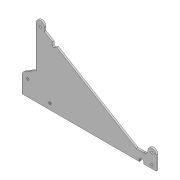
# Autodesk Inventor part: 5linerail
Saved by Autodesk Inventor 2020 (Build 240168000, 168)
## iProperties
Created: 2021-06-11
Part Number: 5linerail
Material: Generic
Document SubType Name: Modeling
Designer: Aidan Lee
Density: 1 g/cm^3
Appearance: Default
Author: Aidan Lee
Autodesk Inventor part; units mm, degrees
ref_plane "YZ Plane" through (0, 0, 0) normal (1, 0, 0) x (0, 1, 0)
ref_plane "XZ Plane" through (0, 0, 0) normal (0, 1, 0) x (-1, 0, 0)
ref_plane "XY Plane" through (0, 0, 0) normal (0, 0, 1) x (1, 0, 0)
sketch "Sketch3" plane through (0, 0, 0) normal (0, 0, 1) x (1, 0, 0)
  circle A0 centre (367.816, 50) radius 50 construction
  line L0 (367.816, 0) -> (512.7041, 0) construction
  line L1 (367.816, 50) -> (512.7041, 50) construction
  line L2 (367.816, 100) -> (512.7041, 100) construction
  line L3 (367.816, 50) -> (342.816, 6.6987) construction
  line L4 (367.816, 50) -> (324.5147, 25) construction
  line L5 (367.816, 50) -> (324.5147, 75) construction
  line L6 (342.816, 93.3013) -> (367.816, 50) construction
  line L7 (392.816, 93.3013) -> (367.816, 50) construction
  line L8 (411.1173, 75) -> (367.816, 50) construction
  line L9 (411.1173, 25) -> (367.816, 50) construction
  line L10 (392.816, 6.6987) -> (367.816, 50) construction
  line L11 (367.816, 0) -> (367.816, 100) construction
  line L12 (417.816, 50) -> (367.816, 50) construction
  line L13 (341.6361, 0) -> (341.6361, 100) construction
  line L14 (315.4561, 0) -> (315.4561, 100) construction
  line L15 (289.2762, 0) -> (289.2762, 100) construction
  line L16 (263.0963, 0) -> (263.0963, 100) construction
  line L17 (236.9163, 0) -> (236.9163, 100) construction
  line L18 (210.7364, 0) -> (210.7364, 100) construction
  line L19 (184.5564, 0) -> (184.5564, 100) construction
  line L20 (158.3765, 0) -> (158.3765, 100) construction
  circle A1 centre (315.4561, 50) radius 50 construction
  circle A2 centre (341.6361, 50) radius 50 construction
  circle A3 centre (289.2762, 50) radius 50 construction
  circle A4 centre (263.0963, 50) radius 50 construction
  circle A5 centre (236.9163, 50) radius 50 construction
  circle A6 centre (210.7364, 50) radius 50 construction
  line L21 (392.816, 6.6987) -> (512.7041, 6.6987) construction
  line L22 (411.1173, 25) -> (512.7041, 25) construction
  line L23 (411.1173, 75) -> (512.7041, 75) construction
  line L24 (411.1173, 75) -> (512.7041, 75) construction
  line L25 (392.816, 93.3013) -> (512.7041, 93.3013) construction
  line L26 (358.7574, 75) -> (339.2762, 50) construction
  line L27 (339.2762, 50) -> (306.3975, 25) construction
  line L28 (306.3975, 25) -> (261.9163, 6.6987) construction
  line L29 (261.9163, 6.6987) -> (210.7364, 0) construction
  line L30 (105.3682, -12.9392) -> (105.3682, 124.4333) construction
  line L31 (21.25, 0) -> (21.25, 12)
  line L32 (35.45, 12) -> (35.45, -11.8433)
  arc A7 (0, 0) -> (6.625, -9.8433) centre (10.625, 0) ccw
  arc A8 (14.625, -9.8433) -> (21.25, 0) centre (10.625, 0) ccw
  line L33 (35.45, -11.8433) -> (14.625, -11.8433)
  line L34 (6.625, -11.8433) -> (-195.0796, -11.8433)
  circle A9 centre (-144.26, 100.8473) radius 12.875 construction
  line L35 (6.625, -11.8433) -> (6.625, -9.8433)
  line L36 (14.625, -11.8433) -> (14.625, -9.8433)
  line L37 (411.1173, 75) -> (158.3765, 75) construction
  line L38 (367.816, 100) -> (158.3765, 100) construction
  line L39 (417.816, 50) -> (158.3765, 50) construction
  line L40 (411.1173, 25) -> (158.3765, 25) construction
  line L41 (392.816, 6.6987) -> (158.3765, 6.6987) construction
  line L42 (392.816, 93.3013) -> (158.3765, 93.3013) construction
  line L43 (358.7574, 75) -> (366.6361, 93.3013) construction
  line L44 (366.6361, 93.3013) -> (367.816, 100) construction
  spline S0 degree 4 poles (-157.0796, 100) (-157.0796, 88.9946) (-147.011, 72.6811) (-131.8577, 48.7932) (-88.4777, 17.6268) (-50.0176, 3.937) (-18.8717, 0) (0, 0) knots 0 0 0 0 0 0.264547 0.457223 0.66608 1 1 1 1 1
  line L45 (-157.0796, 100) -> (-157.0796, 38) construction
  line L46 (0, 0) -> (-157.0796, 0) construction
  line L47 (-144.26, 100.8473) -> (-157.135, 100.8473) construction
  circle A10 centre (-146.4546, 100) radius 10.625 construction
  line L48 (-146.4546, 100) -> (-157.0796, 100) construction
  line L49 (-141.0754, 84.4005) -> (-135.6205, 93.5183) construction
  line L50 (-141.0796, 132.0528) -> (-171.0796, 149.3733) construction
  line L51 (-171.0796, 149.3733) -> (-201.0796, 132.0528) construction
  line L52 (-141.0754, 84.4005) -> (-99.2801, 84.4005) construction
  line L53 (-201.0796, 132.0528) -> (-201.0796, 97.4118) construction
  line L54 (-201.0796, 97.4118) -> (-171.0796, 80.0913) construction
  line L55 (0, 0) -> (-157.0796, 93.9753) construction
  line L56 (-135.6205, 93.5183) -> (-137.3368, 94.5451) construction
  line L57 (-137.3368, 94.5451) -> (-143.2815, 84.6085) construction
  line L58 (-137.3368, 94.5451) -> (-171.0796, 114.7323) construction
  line L59 (-201.0796, 132.0528) -> (-171.0796, 114.7323) construction
  arc A11 (-137.3368, 94.5451) -> (-144.7045, 143.8948) centre (-171.0796, 114.7323) ccw construction
  arc A12 (-142.7917, 85.4273) -> (-147.1443, 147.6882) centre (-171.0796, 114.7323) ccw construction
  line L60 (-171.0796, 80.0913) -> (-171.0796, 35)
  circle A13 centre (-171.0796, 114.7323) radius 2.5 construction
  arc A14 (-167.4345, 120.8251) -> (-174.7248, 108.6394) centre (-171.0796, 114.7323) ccw construction
  line L61 (-167.4345, 120.8251) -> (-157.0796, 114.6302) construction
  line L62 (-171.0796, 80.0913) -> (-171.0796, 106.4587)
  line L63 (-171.0796, 106.4587) -> (-174.7248, 108.6394) construction
  line L64 (-171.0796, 35) -> (-191.5296, 23.1932)
  arc A15 (-191.5296, 23.1932) -> (-195.0796, 17.0444) centre (-187.9796, 17.0444) ccw
  line L65 (-195.0796, 17.0444) -> (-195.0796, -11.8433)
  arc A16 (35.45, 12) -> (21.25, 12) centre (28.35, 12) ccw
  line L66 (-157.0796, 114.6302) -> (-157.0796, 99.9865) construction
  circle A17 centre (-164.0796, 103.4587) radius 2
  line L67 (-171.0796, 103.4587) -> (-157.0796, 103.4587) construction
  circle A18 centre (-185.1284, 15.3983) radius 2
  line L68 (-185.1284, 15.3983) -> (-194.1284, 20.5944) construction
  circle A19 centre (-6, -5.9217) radius 2
  line L69 (-6, -11.8433) -> (-6, 0) construction
  circle A20 centre (28.35, 12) radius 2
  circle A21 centre (28.35, -5.9217) radius 2
  line L70 (-167.4345, 320.8251) -> (-157.0796, 314.6302) construction
  arc A22 (-167.4345, 320.8251) -> (-174.7248, 308.6394) centre (-171.0796, 314.7323) ccw construction
  circle A23 centre (-171.0796, 314.7323) radius 2.5 construction
  line L71 (-171.0796, 280.0913) -> (-171.0796, 306.4587)
  line L72 (-171.0796, 306.4587) -> (-174.7248, 308.6394) construction
  line L73 (-157.0796, 314.6302) -> (-157.0796, 299.9865) construction
  circle A24 centre (-164.0796, 303.4587) radius 2
  spline S1 degree 4 poles (-157.0796, 300) (-157.0796, 288.9946) (-147.0234, 272.6841) (-124.1789, 236.7977) (-70.8039, 208.0704) (-31.8865, 200.2943) (0, 200) knots 0 0 0 0 0 0.264547 0.457223 1 1 1 1 1 construction
  line L74 (-157.0796, 300) -> (-157.0796, 238) construction
  arc A25 (0, 200) -> (6.625, 190.1567) centre (10.625, 200) ccw
  line L75 (35.45, 212) -> (35.45, 188.1567)
  circle A26 centre (28.35, 212) radius 2
  circle A27 centre (28.35, 194.0783) radius 2
  arc A28 (35.45, 212) -> (21.25, 212) centre (28.35, 212) ccw
  line L76 (21.25, 200) -> (21.25, 212)
  line L77 (35.45, 188.1567) -> (14.625, 188.1567)
  arc A29 (14.625, 190.1567) -> (21.25, 200) centre (10.625, 200) ccw
  line L78 (14.625, 188.1567) -> (14.625, 190.1567)
  line L79 (-185.1284, 215.3983) -> (-194.1284, 220.5944) construction
  arc A30 (-191.5296, 223.1932) -> (-195.0796, 217.0444) centre (-187.9796, 217.0444) ccw
  line L80 (-195.0796, 217.0444) -> (-195.0796, 188.1567)
  line L81 (-171.0796, 235) -> (-191.5296, 223.1932)
  circle A31 centre (-185.1284, 215.3983) radius 2
  line L82 (-171.0796, 280.0913) -> (-171.0796, 235)
  line L83 (6.625, 188.1567) -> (-195.0796, 188.1567)
  line L84 (6.625, 188.1567) -> (6.625, 190.1567)
  line L85 (-137.3368, 294.5451) -> (-143.2815, 284.6085) construction
  line L86 (-141.0754, 284.4005) -> (-135.6205, 293.5183) construction
  line L87 (0, 200) -> (-157.0796, 293.9753)
  line L88 (-167.4345, 520.8251) -> (-157.0796, 514.6302) construction
  arc A32 (-167.4345, 520.8251) -> (-174.7248, 508.6394) centre (-171.0796, 514.7323) ccw construction
  circle A33 centre (-171.0796, 514.7323) radius 2.5 construction
  line L89 (-171.0796, 480.0913) -> (-171.0796, 506.4587)
  line L90 (-171.0796, 506.4587) -> (-174.7248, 508.6394) construction
  line L91 (-157.0796, 514.6302) -> (-157.0796, 499.9865) construction
  circle A34 centre (-164.0796, 503.4587) radius 2
  spline S2 degree 4 poles (-157.0796, 500) (-157.0796, 488.9946) (-147.0234, 472.6841) (-124.1789, 436.7977) (-70.8039, 408.0704) (-31.8865, 400.2943) (0, 400) knots 0 0 0 0 0 0.264547 0.457223 1 1 1 1 1 construction
  line L92 (-157.0796, 500) -> (-157.0796, 438)
  arc A35 (0, 400) -> (6.625, 390.1567) centre (10.625, 400) ccw
  line L93 (35.45, 412) -> (35.45, 388.1567)
  circle A36 centre (28.35, 412) radius 2
  circle A37 centre (28.35, 394.0783) radius 2
  arc A38 (35.45, 412) -> (21.25, 412) centre (28.35, 412) ccw
  line L94 (21.25, 400) -> (21.25, 412)
  line L95 (35.45, 388.1567) -> (14.625, 388.1567)
  arc A39 (14.625, 390.1567) -> (21.25, 400) centre (10.625, 400) ccw
  line L96 (14.625, 388.1567) -> (14.625, 390.1567)
  line L97 (-185.1284, 415.3983) -> (-194.1284, 420.5944) construction
  arc A40 (-191.5296, 423.1932) -> (-195.0796, 417.0444) centre (-187.9796, 417.0444) ccw
  line L98 (-195.0796, 417.0444) -> (-195.0796, 388.1567)
  line L99 (-171.0796, 435) -> (-191.5296, 423.1932)
  circle A41 centre (-185.1284, 415.3983) radius 2
  line L100 (-171.0796, 480.0913) -> (-171.0796, 435)
  line L101 (6.625, 388.1567) -> (-195.0796, 388.1567)
  line L102 (6.625, 388.1567) -> (6.625, 390.1567)
  line L103 (-137.3368, 494.5451) -> (-143.2815, 484.6085) construction
  line L104 (-141.0754, 484.4005) -> (-135.6205, 493.5183) construction
  line L105 (0, 400) -> (-157.0796, 493.9753) construction
  line L106 (-467.4345, 120.8251) -> (-457.0796, 114.6302) construction
  arc A42 (-467.4345, 120.8251) -> (-474.7248, 108.6394) centre (-471.0796, 114.7323) ccw construction
  circle A43 centre (-471.0796, 114.7323) radius 2.5 construction
  line L107 (-471.0796, 80.0913) -> (-471.0796, 106.4587)
  line L108 (-471.0796, 106.4587) -> (-474.7248, 108.6394) construction
  line L109 (-457.0796, 114.6302) -> (-457.0796, 99.9865) construction
  circle A44 centre (-464.0796, 103.4587) radius 2
  spline S3 degree 4 poles (-457.0796, 100) (-457.0796, 88.9946) (-447.0234, 72.6841) (-424.1789, 36.7977) (-370.8039, 8.0704) (-331.8865, 0.2943) (-300, 0) knots 0 0 0 0 0 0.264547 0.457223 1 1 1 1 1 construction
  line L110 (-457.0796, 100) -> (-457.0796, 38) construction
  arc A45 (-300, 0) -> (-293.375, -9.8433) centre (-289.375, 0) ccw construction
  line L111 (-264.55, 12) -> (-264.55, -11.8433)
  circle A46 centre (-271.65, 12) radius 2
  circle A47 centre (-271.65, -5.9217) radius 2
  arc A48 (-264.55, 12) -> (-278.75, 12) centre (-271.65, 12) ccw
  line L112 (-278.75, 0) -> (-278.75, 12) construction
  line L113 (-264.55, -11.8433) -> (-285.375, -11.8433)
  arc A49 (-285.375, -9.8433) -> (-278.75, 0) centre (-289.375, 0) ccw construction
  line L114 (-285.375, -11.8433) -> (-285.375, -9.8433) construction
  line L115 (-485.1284, 15.3983) -> (-494.1284, 20.5944) construction
  arc A50 (-491.5296, 23.1932) -> (-495.0796, 17.0444) centre (-487.9796, 17.0444) ccw
  line L116 (-495.0796, 17.0444) -> (-495.0796, -11.8433)
  line L117 (-471.0796, 35) -> (-491.5296, 23.1932)
  circle A51 centre (-485.1284, 15.3983) radius 2
  line L118 (-471.0796, 80.0913) -> (-471.0796, 35)
  line L119 (-293.375, -11.8433) -> (-495.0796, -11.8433)
  line L120 (-293.375, -11.8433) -> (-293.375, -9.8433) construction
  line L121 (-437.3368, 94.5451) -> (-443.2815, 84.6085) construction
  line L122 (-441.0754, 84.4005) -> (-435.6205, 93.5183) construction
  line L123 (-300, 0) -> (-457.0796, 93.9753) construction
  line L124 (-467.4345, 320.8251) -> (-457.0796, 314.6302) construction
  arc A52 (-467.4345, 320.8251) -> (-474.7248, 308.6394) centre (-471.0796, 314.7323) ccw construction
  circle A53 centre (-471.0796, 314.7323) radius 2.5 construction
  line L125 (-471.0796, 280.0913) -> (-471.0796, 306.4587)
  line L126 (-471.0796, 306.4587) -> (-474.7248, 308.6394) construction
  line L127 (-457.0796, 314.6302) -> (-457.0796, 299.9865) construction
  circle A54 centre (-464.0796, 303.4587) radius 2
  spline S4 degree 4 poles (-457.0796, 300) (-457.0796, 288.9946) (-447.0234, 272.6841) (-424.1789, 236.7977) (-370.8039, 208.0704) (-331.8865, 200.2943) (-300, 200) knots 0 0 0 0 0 0.264547 0.457223 1 1 1 1 1 construction
  line L128 (-457.0796, 300) -> (-457.0796, 238) construction
  arc A55 (-300, 200) -> (-293.375, 190.1567) centre (-289.375, 200) ccw construction
  line L129 (-264.55, 212) -> (-264.55, 188.1567)
  circle A56 centre (-271.65, 212) radius 2
  circle A57 centre (-271.65, 194.0783) radius 2
  arc A58 (-264.55, 212) -> (-278.75, 212) centre (-271.65, 212) ccw
  line L130 (-278.75, 200) -> (-278.75, 212) construction
  line L131 (-264.55, 188.1567) -> (-285.375, 188.1567)
  arc A59 (-285.375, 190.1567) -> (-278.75, 200) centre (-289.375, 200) ccw construction
  line L132 (-285.375, 188.1567) -> (-285.375, 190.1567) construction
  line L133 (-485.1284, 215.3983) -> (-494.1284, 220.5944) construction
  arc A60 (-491.5296, 223.1932) -> (-495.0796, 217.0444) centre (-487.9796, 217.0444) ccw
  line L134 (-495.0796, 217.0444) -> (-495.0796, 188.1567)
  line L135 (-471.0796, 235) -> (-491.5296, 223.1932)
  circle A61 centre (-485.1284, 215.3983) radius 2
  line L136 (-471.0796, 280.0913) -> (-471.0796, 235)
  line L137 (-293.375, 188.1567) -> (-495.0796, 188.1567)
  line L138 (-293.375, 188.1567) -> (-293.375, 190.1567) construction
  line L139 (-437.3368, 294.5451) -> (-443.2815, 284.6085) construction
  line L140 (-441.0754, 284.4005) -> (-435.6205, 293.5183) construction
  line L141 (-300, 200) -> (-457.0796, 293.9753) construction
  line L142 (-467.4345, 520.8251) -> (-457.0796, 514.6302)
  arc A62 (-467.4345, 520.8251) -> (-474.7248, 508.6394) centre (-471.0796, 514.7323) ccw
  circle A63 centre (-471.0796, 514.7323) radius 2.5
  line L143 (-471.0796, 480.0913) -> (-471.0796, 506.4587)
  line L144 (-471.0796, 506.4587) -> (-474.7248, 508.6394)
  line L145 (-457.0796, 514.6302) -> (-457.0796, 499.9865)
  circle A64 centre (-464.0796, 503.4587) radius 2
  spline S5 degree 4 poles (-457.0796, 500) (-457.0796, 488.9946) (-447.0234, 472.6841) (-424.1789, 436.7977) (-370.8039, 408.0704) (-331.8865, 400.2943) (-300, 400) knots 0 0 0 0 0 0.264547 0.457223 1 1 1 1 1 construction
  line L146 (-457.0796, 500) -> (-457.0796, 438) construction
  arc A65 (-300, 400) -> (-293.375, 390.1567) centre (-289.375, 400) ccw construction
  line L147 (-264.55, 412) -> (-264.55, 388.1567) construction
  circle A66 centre (-271.65, 412) radius 2
  circle A67 centre (-271.65, 394.0783) radius 2
  arc A68 (-264.55, 412) -> (-278.75, 412) centre (-271.65, 412) ccw
  line L148 (-278.75, 400) -> (-278.75, 412) construction
  line L149 (-264.55, 388.1567) -> (-285.375, 388.1567)
  arc A69 (-285.375, 390.1567) -> (-278.75, 400) centre (-289.375, 400) ccw construction
  line L150 (-285.375, 388.1567) -> (-285.375, 390.1567) construction
  line L151 (-485.1284, 415.3983) -> (-494.1284, 420.5944) construction
  arc A70 (-491.5296, 423.1932) -> (-495.0796, 417.0444) centre (-487.9796, 417.0444) ccw
  line L152 (-495.0796, 417.0444) -> (-495.0796, 388.1567) construction
  line L153 (-471.0796, 435) -> (-491.5296, 423.1932)
  circle A71 centre (-485.1284, 415.3983) radius 2
  line L154 (-471.0796, 480.0913) -> (-471.0796, 435)
  line L155 (-293.375, 388.1567) -> (-495.0796, 388.1567)
  line L156 (-293.375, 388.1567) -> (-293.375, 390.1567) construction
  line L157 (-437.3368, 494.5451) -> (-443.2815, 484.6085) construction
  line L158 (-441.0754, 484.4005) -> (-435.6205, 493.5183) construction
  line L159 (-300, 400) -> (-457.0796, 493.9753) construction
  line L160 (-435.4304, 87.048) -> (-430.3073, 83.9831)
  line L161 (-430.3073, 83.9831) -> (-430.3073, 78.0131)
  line L162 (-457.0796, 100) -> (-443.128, 91.6532)
  line L163 (-443.2208, 85.684) -> (-443.128, 91.6532)
  line L164 (-440.6463, 84.1438) -> (-435.4304, 87.048)
  line L165 (-440.6463, 84.1438) -> (-443.2208, 85.684)
  line L166 (-430.3073, 78.0131) -> (-436.0283, 74.7101)
  line L167 (-436.0283, 74.7101) -> (-436.0283, 68.1041)
  spline S6 degree 4 poles (-439.3753, 72.7777) (-420.1522, 45.3403) (-398.6357, 22.4496) (-337.1208, 4.2654) (-300, 5.1701) knots 0 0 0 0 0 1 1 1 1 1
  line L168 (-293.375, -11.8433) -> (-285.375, -11.8433)
  line L169 (-157.0796, 293.9753) -> (-157.0796, 300)
  line L170 (-293.375, 188.1567) -> (-285.375, 188.1567)
  arc A72 (-157.0796, 438) -> (-119.0796, 400) centre (-119.0796, 438) ccw
  line L171 (-119.0796, 400) -> (0, 400)
  line L172 (-457.0796, 500) -> (-457.0796, 438) construction
  line L173 (-419.0796, 400) -> (-300, 400) construction
  arc A73 (-457.0796, 438) -> (-419.0796, 400) centre (-419.0796, 438) ccw construction
  line L174 (-457.0796, 300) -> (-443.128, 291.6532)
  line L175 (-443.2208, 285.684) -> (-443.128, 291.6532)
  line L176 (-440.6463, 284.1438) -> (-443.2208, 285.684)
  line L177 (-440.6463, 284.1438) -> (-435.4304, 287.048)
  line L178 (-435.4304, 287.048) -> (-430.3073, 283.9831)
  line L179 (-430.3073, 283.9831) -> (-430.3073, 278.0131) construction
  line L180 (-430.3073, 278.0131) -> (-436.0283, 274.7101) construction
  line L181 (-457.0796, 500) -> (-443.128, 491.6532)
  line L182 (-443.2208, 485.684) -> (-443.128, 491.6532)
  line L183 (-440.6463, 484.1438) -> (-443.2208, 485.684)
  line L184 (-440.6463, 484.1438) -> (-435.4304, 487.048)
  line L185 (-435.4304, 487.048) -> (-430.3073, 483.9831)
  line L186 (-430.3073, 483.9831) -> (-430.3073, 478.0131)
  line L187 (-430.3073, 478.0131) -> (-436.0283, 474.7101)
  line L188 (-430.3073, 283.9831) -> (-298.5715, 205.1701)
  line L189 (-293.375, 388.1567) -> (-285.375, 388.1567)
  line L190 (-300, 5.1701) -> (-285.5799, 5.1701)
  arc A74 (-285.5799, 5.1701) -> (-278.75, 12) centre (-285.5799, 12) ccw
  line L191 (-298.5715, 205.1701) -> (-285.5799, 205.1701)
  arc A75 (-285.5799, 205.1701) -> (-278.75, 212) centre (-285.5799, 212) ccw
  line L192 (-436.0283, 474.7101) -> (-451.9095, 465.5411)
  line L193 (-451.9095, 465.5411) -> (-451.9095, 438)
  arc A76 (-451.9095, 438) -> (-419.0796, 405.1701) centre (-419.0796, 438) ccw
  line L194 (-419.0796, 405.1701) -> (-285.5799, 405.1701)
  arc A77 (-285.5799, 405.1701) -> (-278.75, 412) centre (-285.5799, 412) ccw
  line L195 (-495.0796, 388.1567) -> (-514.2796, 388.1567)
  line L196 (-514.2796, 388.1567) -> (-514.2796, 392.1567)
  line L197 (-514.2796, 392.1567) -> (-498.0796, 392.1567)
  arc A78 (-498.0796, 392.1567) -> (-495.0796, 395.1567) centre (-498.0796, 395.1567) ccw
  line L198 (-495.0796, 395.1567) -> (-495.0796, 417.0444)
  line L199 (-499.0796, 388.1567) -> (-510.2796, 388.1567) construction
  line L200 (-510.2796, 388.1567) -> (-510.2796, 392.1567) construction
  line L201 (-510.2796, 392.1567) -> (-499.0796, 392.1567) construction
  line L202 (-499.0796, 392.1567) -> (-499.0796, 388.1567) construction
  line L203 (-499.0796, 388.1567) -> (-510.2796, 392.1567) construction
  line L204 (-510.2796, 388.1567) -> (-499.0796, 392.1567) construction
  arc A79 (-600, 200) -> (-593.375, 190.1567) centre (-589.375, 200) ccw construction
  line L205 (-564.55, 212) -> (-564.55, 188.1567) construction
  circle A80 centre (-571.65, 212) radius 2
  circle A81 centre (-571.65, 194.0783) radius 2
  arc A82 (-564.55, 212) -> (-578.75, 212) centre (-571.65, 212) ccw
  line L206 (-578.75, 200) -> (-578.75, 212) construction
  line L207 (-564.55, 188.1567) -> (-585.375, 188.1567)
  arc A83 (-585.375, 190.1567) -> (-578.75, 200) centre (-589.375, 200) ccw construction
  line L208 (-585.375, 188.1567) -> (-585.375, 190.1567) construction
  line L209 (-593.375, 188.1567) -> (-593.375, 190.1567) construction
  arc A84 (-585.5799, 205.1701) -> (-578.75, 212) centre (-585.5799, 212) ccw
  line L210 (-593.375, 188.1567) -> (-585.375, 188.1567)
  line L211 (-598.5715, 205.1701) -> (-585.5799, 205.1701)
  arc A85 (-791.5296, 223.1932) -> (-795.0796, 217.0444) centre (-787.9796, 217.0444) ccw
  line L212 (-785.1284, 215.3983) -> (-794.1284, 220.5944) construction
  circle A86 centre (-785.1284, 215.3983) radius 2
  line L213 (-771.0796, 235) -> (-791.5296, 223.1932)
  line L214 (-795.0796, 217.0444) -> (-795.0796, 188.1567) construction
  line L215 (-730.3073, 278.0131) -> (-736.0283, 274.7101) construction
  line L216 (-757.0796, 300) -> (-757.0796, 238) construction
  line L217 (-730.3073, 283.9831) -> (-730.3073, 278.0131) construction
  line L218 (-730.3073, 283.9831) -> (-598.5715, 205.1701)
  line L219 (-600, 200) -> (-757.0796, 293.9753) construction
  spline S7 degree 4 poles (-757.0796, 300) (-757.0796, 288.9946) (-747.0234, 272.6841) (-724.1789, 236.7977) (-670.8039, 208.0704) (-631.8865, 200.2943) (-600, 200) knots 0 0 0 0 0 0.264547 0.457223 1 1 1 1 1 construction
  line L220 (-593.375, 188.1567) -> (-795.0796, 188.1567)
  line L221 (-771.0796, 280.0913) -> (-771.0796, 235)
  line L222 (-757.0796, 300) -> (-743.128, 291.6532)
  line L223 (-743.2208, 285.684) -> (-743.128, 291.6532)
  line L224 (-740.6463, 284.1438) -> (-743.2208, 285.684)
  line L225 (-737.3368, 294.5451) -> (-743.2815, 284.6085) construction
  line L226 (-741.0754, 284.4005) -> (-735.6205, 293.5183) construction
  line L227 (-740.6463, 284.1438) -> (-735.4304, 287.048)
  line L228 (-735.4304, 287.048) -> (-730.3073, 283.9831)
  line L229 (-767.4345, 320.8251) -> (-757.0796, 314.6302)
  line L230 (-771.0796, 280.0913) -> (-771.0796, 306.4587)
  line L231 (-757.0796, 314.6302) -> (-757.0796, 299.9865)
  circle A87 centre (-764.0796, 303.4587) radius 2
  line L232 (-771.0796, 306.4587) -> (-774.7248, 308.6394)
  circle A88 centre (-771.0796, 314.7323) radius 2.5
  arc A89 (-767.4345, 320.8251) -> (-774.7248, 308.6394) centre (-771.0796, 314.7323) ccw
  line L233 (-795.0796, 188.1567) -> (-814.2796, 188.1567)
  line L234 (-814.2796, 188.1567) -> (-814.2796, 192.1567)
  line L235 (-814.2796, 192.1567) -> (-798.0796, 192.1567)
  arc A90 (-798.0796, 192.1567) -> (-795.0796, 195.1567) centre (-798.0796, 195.1567) ccw
  line L236 (-795.0796, 195.1567) -> (-795.0796, 217.0444)
  line L237 (-799.0796, 188.1567) -> (-810.2796, 188.1567) construction
  line L238 (-810.2796, 188.1567) -> (-810.2796, 192.1567) construction
  line L239 (-810.2796, 192.1567) -> (-799.0796, 192.1567) construction
  line L240 (-799.0796, 192.1567) -> (-799.0796, 188.1567) construction
  line L241 (-799.0796, 188.1567) -> (-810.2796, 192.1567) construction
  line L242 (-810.2796, 188.1567) -> (-799.0796, 192.1567) construction
  line L243 (-495.0796, 587.6927) -> (-264.55, 587.6927) construction
  line L244 (-379.8148, 587.6927) -> (-379.8148, 614.3146) construction
  line L245 (-795.0796, 438) -> (-564.55, 438) construction
  line L246 (-679.8148, 438) -> (-679.8148, 492.8294) construction
  arc A91 (-564.55, 195.1567) -> (-561.55, 192.1567) centre (-561.55, 195.1567) ccw
  line L247 (-545.35, 192.1567) -> (-561.55, 192.1567)
  line L248 (-545.35, 188.1567) -> (-545.35, 192.1567)
  line L249 (-560.55, 192.1567) -> (-560.55, 188.1567) construction
  line L250 (-560.55, 188.1567) -> (-549.35, 188.1567) construction
  line L251 (-564.55, 188.1567) -> (-545.35, 188.1567)
  line L252 (-549.35, 188.1567) -> (-549.35, 192.1567) construction
  line L253 (-549.35, 192.1567) -> (-560.55, 192.1567) construction
  line L254 (-560.55, 188.1567) -> (-549.35, 192.1567) construction
  line L255 (-549.35, 188.1567) -> (-560.55, 192.1567) construction
  line L256 (-564.55, 195.1567) -> (-564.55, 212)
  circle A92 centre (-147.0796, 398.1567) radius 2
  circle A93 centre (-147.0796, 198.1567) radius 2
  circle A94 centre (-147.0796, -1.8433) radius 2
  circle A95 centre (-447.0796, 398.1567) radius 2
  circle A96 centre (-447.0796, 198.1567) radius 2
  circle A97 centre (-447.0796, -1.8433) radius 2
  circle A98 centre (-747.0796, 398.1567) radius 2 construction
  circle A99 centre (-747.0796, 198.1567) radius 2
  circle A100 centre (-747.0796, -1.8433) radius 2 construction
  line L257 (-264.55, 388.1567) -> (-245.35, 388.1567)
  line L258 (-245.35, 388.1567) -> (-245.35, 392.1567)
  line L259 (-245.35, 392.1567) -> (-261.55, 392.1567)
  arc A101 (-264.55, 395.1567) -> (-261.55, 392.1567) centre (-261.55, 395.1567) ccw
  line L260 (-260.55, 388.1567) -> (-249.35, 388.1567) construction
  line L261 (-249.35, 388.1567) -> (-249.35, 392.1567) construction
  line L262 (-249.35, 392.1567) -> (-260.55, 392.1567) construction
  line L263 (-260.55, 392.1567) -> (-260.55, 388.1567) construction
  line L264 (-260.55, 388.1567) -> (-249.35, 392.1567) construction
  line L265 (-249.35, 388.1567) -> (-260.55, 392.1567) construction
  line L266 (-264.55, 412) -> (-264.55, 395.1567)
  arc A102 (-157.0796, 106.4587) -> (-171.0796, 106.4587) centre (-164.0796, 106.4587) ccw
  line L267 (-157.0796, 106.4587) -> (-157.0796, 100)
  arc A103 (-157.0796, 306.4587) -> (-171.0796, 306.4587) centre (-164.0796, 306.4587) ccw
  line L268 (-157.0796, 306.4587) -> (-157.0796, 300)
  arc A104 (-157.0796, 506.4587) -> (-171.0796, 506.4587) centre (-164.0796, 506.4587) ccw
  line L269 (-157.0796, 506.4587) -> (-157.0796, 500)
  arc A105 (-457.0796, 106.4587) -> (-471.0796, 106.4587) centre (-464.0796, 106.4587) ccw
  line L270 (-457.0796, 106.4587) -> (-457.0796, 100)
  arc A106 (-457.0796, 306.4587) -> (-471.0796, 306.4587) centre (-464.0796, 306.4587) ccw
  line L271 (-457.0796, 306.4587) -> (-457.0796, 300)
  arc A107 (-457.0796, 506.4587) -> (-471.0796, 506.4587) centre (-464.0796, 506.4587) ccw construction
  line L272 (-457.0796, 506.4587) -> (-457.0796, 500) construction
  point P0 (158.3765, 0)
  point P1 (-148.021, 75)
  point P2 (-128.5398, 50)
  point P3 (-95.6611, 25)
  point P4 (-51.1799, 6.6987)
  point P5 (-155.8997, 93.3013)
  point P6 (-148.021, 275)
  point P7 (-128.5398, 250)
  point P8 (-95.6611, 225)
  point P9 (-51.1799, 206.6987)
  point P10 (-157.0796, 303.4587)
  point P11 (-157.0796, 200)
  point P12 (-171.0796, 303.4587)
  point P13 (-6, 188.1567)
  point P14 (-142.7917, 285.4273)
  point P15 (-148.021, 475)
  point P16 (-128.5398, 450)
  point P17 (-95.6611, 425)
  point P18 (-51.1799, 406.6987)
  point P19 (-157.0796, 503.4587)
  point P20 (-157.0796, 400)
  point P21 (-171.0796, 503.4587)
  point P22 (-6, 388.1567)
  point P23 (-142.7917, 485.4273)
  point P24 (-448.021, 75)
  point P25 (-428.5398, 50)
  point P26 (-395.6611, 25)
  point P27 (-351.1799, 6.6987)
  point P28 (-457.0796, 103.4587)
  point P29 (-457.0796, 0)
  point P30 (-471.0796, 103.4587)
  point P31 (-306, -11.8433)
  point P32 (-442.7917, 85.4273)
  point P33 (-448.021, 275)
  point P34 (-428.5398, 250)
  point P35 (-395.6611, 225)
  point P36 (-351.1799, 206.6987)
  point P37 (-457.0796, 303.4587)
  point P38 (-457.0796, 200)
  point P39 (-471.0796, 303.4587)
  point P40 (-306, 188.1567)
  point P41 (-442.7917, 285.4273)
  point P42 (-448.021, 475)
  point P43 (-428.5398, 450)
  point P44 (-395.6611, 425)
  point P45 (-351.1799, 406.6987)
  point P46 (-457.0796, 503.4587)
  point P47 (-457.0796, 400)
  point P48 (-471.0796, 503.4587)
  point P49 (-306, 388.1567)
  point P50 (-442.7917, 485.4273)
  point P51 (-421.2258, 50.7726)
  point P52 (-392.6255, 29.6644)
  point P53 (-346.6709, 11.6004)
  point P54 (-436.0267, 68.102)
  point P55 (-457.0796, 503.4587)
  point P56 (-504.6796, 390.1567)
  point P57 (-606, 188.1567)
  point P58 (-757.0796, 200)
  point P59 (-748.021, 275)
  point P60 (-728.5398, 250)
  point P61 (-757.0796, 303.4587)
  point P62 (-695.6611, 225)
  point P63 (-651.1799, 206.6987)
  point P64 (-742.7917, 285.4273)
  point P65 (-771.0796, 303.4587)
  point P66 (-804.6796, 190.1567)
  point P67 (-564.55, 188.1567)
  point P68 (-554.95, 190.1567)
  point P69 (-254.95, 390.1567)
  point P70 (-278.75, 12)
  dimension "d43" = 25.75
  dimension "diameter" = 100
  dimension "d8" = 26.1799
  dimension "d14" = 30
  dimension "d15" = 30
  dimension "d16" = 30
  dimension "d32" = 10.625
  dimension "d47" = 8
  dimension "d49" = 2
  dimension "d53" = 21.25
  dimension "d62" = 20.825
  dimension "d123" = 120
  dimension "d126" = 59.109
  dimension "d137" = 2
  dimension "d138" = 90
  dimension "d139" = 90
  dimension "d141" = 7.1
  dimension "d142" = 14
  dimension "d143" = 7.1
  dimension "d144" = 12
  dimension "d145" = 5
  dimension "d146" = 35
  dimension "d147" = 24
  dimension "hole" = 4
  dimension "d155" = 4
  dimension "d156" = 9
  dimension "d157" = 4
  dimension "d158" = 6
  dimension "d159" = 4
  dimension "d160" = 4
  dimension "d241" = 120.891
  dimension "d244" = 120
  dimension "d245" = 30
  dimension "d246" = 3
  dimension "d249" = 200
  dimension "d252" = 300
  dimension "d255" = 120
  dimension "d256" = 5.1701
  dimension "d259" = 0.5
  dimension "d260" = 0.5
  dimension "d261" = 120
  dimension "d262" = 120
  dimension "d264" = 5.1701
  dimension "d265" = 38
  dimension "d268" = 300
  dimension "d275" = 200
  dimension "d288" = 5.1701
  dimension "d289" = 5.1701
  dimension "d290" = 5.1701
  dimension "d291" = 5.1701
  dimension "d292" = 11.2
  dimension "d293" = 4
  dimension "d294" = 4
  dimension "d296" = 3
  dimension "d299" = 300
  dimension "d324" = 11.2
  dimension "d325" = 4
  dimension "d326" = 4
  dimension "d328" = 3
  dimension "d330" = 4
  dimension "d331" = 10
  dimension "d332" = 10
  dimension "d335" = 200
  dimension "d338" = 300
  dimension "d341" = 7.1
  dimension "d342" = 4.6
  constraints: 544 end point, 121 point on circle, 105 centre point, 64 point on line, 40 horizontal, 36 coincident, 30 symmetric about line, 21 tangent, 21 vertical, 19 midpoint, 18 horizontal alignment, 17 perpendicular, 15 vertical alignment, 13 parallel, 8 collinear, 8 equal length, 1 concentric, 656 other
  measures "d8" distance of L11.start L13.start
  measures "d14" angle of L6 L11
  measures "d15" angle of L11 L7
  measures "d16" angle of L9 L12
  measures "d32" radius of A7
  measures "d47" distance between parallel lines of L35 L36
  measures "d49" distance of L34.start L35.end
  measures "d53" diameter of A10
  measures "d62" distance between parallel lines of L32 L36
  measures "d123" angle of L50 L51
  measures "d126" angle of L49 L52
  measures "d137" distance between parallel lines of L57 L49
  measures "d138" angle of L55 L57
  measures "d139" angle of L57 L58
  measures "d141" radius of A15
  measures "d142" distance between parallel lines of L60 L45
  measures "d143" radius of A16
  measures "d144" vertical distance of A16.centre point (0, 0)
  measures "d145" diameter of A13
  measures "d146" vertical distance of L60.end point (0, 0)
  measures "d147" distance between parallel lines of L60 L65
  measures "hole" diameter of A17
  measures "d155" diameter of A18
  measures "d156" horizontal distance of L68.start L68.end
  measures "d157" diameter of A19
  measures "d158" distance from line of point (0, 0) L69
  measures "d159" diameter of A20
  measures "d160" diameter of A21
  measures "d241" angle of L45 L58
  measures "d244" angle of L60 L54
  measures "d245" horizontal distance of L53.end L54.end
  measures "d246" vertical distance of L62.end A17.centre
  measures "d249" distance of L61.start L70.start
  measures "d252" distance of L61.start L106.start
  measures "d255" angle of L167 L166
  measures "d256" distance between parallel lines of L123 L162
  measures "d259" distance from line of L165.start L122
  measures "d260" distance from line of L163.start L121
  measures "d261" angle of L163 L162
  measures "d262" angle of L160 L164
  measures "d264" distance between parallel lines of L123 L160
  measures "d265" radius of A72
  measures "d268" distance of L92.start L172.start
  measures "d275" distance of L162.start L174.start
  measures "d288" distance of L190.start L123.start
  measures "d289" distance from line of L141.start L191
  measures "d290" distance between parallel lines of L173 L194
  measures "d291" distance between parallel lines of L146 L193
  measures "d292" distance between parallel lines of L200 L202
  measures "d293" distance between parallel lines of L196 L200
  measures "d294" distance of L195.end L196.end
  measures "d296" radius of A78
  measures "d299" distance of L135.end L213.end
  measures "d324" distance between parallel lines of L238 L240
  measures "d325" distance between parallel lines of L234 L238
  measures "d326" distance of L234.start L235.start
  measures "d328" radius of A90
  measures "d330" diameter of A92
  measures "d331" distance from line of L101 A92.centre
  measures "d332" distance from line of A92.centre L92
  measures "d335" distance of A92.centre A93.centre
  measures "d338" distance of A92.centre A95.centre
  measures "d341" radius of A14
  measures "d342" radial gap between concentric circles of A14 A13
sketch "Sketch5" plane through (0, 0, 0) normal (0, 0, 1) x (1, 0, 0)
  circle A0 centre (-171.0796, 114.7323) radius 2
  arc A1 (-168.5126, 119.023) -> (-173.6466, 110.4415) centre (-171.0796, 114.7323) ccw construction
  line L0 (-173.6466, 110.4415) -> (-168.5126, 119.023) construction
  line L1 (-137.3368, 94.5451) -> (-171.0796, 114.7323) construction
  line L2 (-137.3368, 94.5451) -> (-143.2815, 84.6085) construction
  line L3 (-141.0754, 84.4005) -> (-135.6205, 93.5183) construction
  line L4 (-142.7917, 85.4273) -> (-141.0754, 84.4005) construction
  line L5 (-173.6466, 110.4415) -> (-138.1875, 89.2276) construction
  line L6 (-138.1875, 89.2276) -> (-133.0535, 97.8091)
  line L7 (-133.0535, 97.8091) -> (-168.5126, 119.023) construction
  line L8 (-159.6382, 113.7138) -> (-159.6382, 107.8873)
  line L9 (-159.6382, 107.8873) -> (-145.3456, 99.3365)
  line L10 (-133.0535, 97.8091) -> (-140.2116, 102.0915)
  line L11 (-152.4919, 103.6119) -> (-153.6918, 101.6062)
  line L12 (-140.2116, 102.0915) -> (-145.3456, 99.3365)
  line L13 (-159.6382, 113.7138) -> (-168.5126, 119.023)
  line L14 (-135.6205, 93.5183) -> (-169.3633, 113.7055) construction
  line L15 (-168.5126, 119.023) -> (-189.9664, 131.858)
  arc A2 (-189.9664, 131.858) -> (-195.1004, 123.2766) centre (-192.5334, 127.5673) ccw
  line L16 (-195.1004, 123.2766) -> (-173.6466, 110.4415)
  line L17 (-142.7917, 85.4273) -> (-141.0754, 84.4005)
  line L18 (-141.0754, 84.4005) -> (-138.1875, 89.2276)
  line L19 (-142.7917, 85.4273) -> (-142.6907, 91.9217)
  line L20 (-142.6907, 91.9217) -> (-173.6466, 110.4415)
  arc A3 (-141.0754, 84.4005) -> (-138.014, 141.6941) centre (-171.0796, 114.7323) ccw construction
  point P0 (0, 0)
  dimension "d346" = 4
  dimension "d347" = 3
  dimension "d356" = 25
  dimension "d357" = 120
  constraints: 36 end point, 9 point on line, 7 perpendicular, 6 point on circle, 4 midpoint, 3 centre point, 3 coincident, 3 collinear, 2 tangent, 1 symmetric about line, 1 vertical, 3 other
  measures "d356" distance from line of L15.end L0
  measures "d357" angle of L5 L19
extrude "Extrusion7" add sketch "Sketch3" along normal blind 3 contours L125 A106 L271 L174 L175 L176 L177 L178 L188 L191 A75 A58 L129 L131 L170 L137 L134 A60 L135 L136
sketch "Sketch6" plane through (0, 0, 0) normal (0, 0, -1) x (-1, 0, 0)
  line L0 (285.375, 188.1567) -> (285.375, 190.1567) projected
  line L1 (293.375, 188.1567) -> (293.375, 190.1567) projected
  arc A0 (293.375, 190.1567) -> (285.375, 190.1567) centre (289.375, 190.1567) ccw
  line L2 (285.375, 188.1567) -> (293.375, 188.1567)
  line L3 (495.0796, 188.1567) -> (264.55, 188.1567) projected
  point P0 (0, 0)
  constraints: 2 end point, 2 point on circle, 1 centre point, 1 collinear, 1 horizontal alignment
extrude "Extrusion8" cut sketch "Sketch6" against normal through all
body "Solid7"
